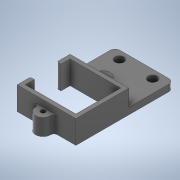
# Autodesk Inventor part: SocketMount
Saved by Autodesk Inventor 2020.2 (Build 242310000, 310)
## iProperties
Created: 2020-08-26
Part Number: SocketMount
Material: Generic
Document SubType Name: Modeling
Designer: JK
Density: 1 g/cm^3
Appearance: Smooth - Black
Author: JK
Autodesk Inventor part; units mm, degrees
ref_plane "YZ Plane" through (0, 0, 0) normal (1, 0, 0) x (0, 1, 0)
ref_plane "XZ Plane" through (0, 0, 0) normal (0, 1, 0) x (-1, 0, 0)
ref_plane "XY Plane" through (0, 0, 0) normal (0, 0, 1) x (1, 0, 0)
sketch "Sketch1" plane through (0, 0, 0) normal (0, 1, 0) x (-1, 0, 0)
  line L0 (-26.4056, 15.9) -> (8.8944, 15.9)
  line L1 (8.8944, 15.9) -> (8.8944, -15.9)
  line L2 (8.8944, -15.9) -> (-26.4056, -15.9)
  line L3 (-26.4056, -15.9) -> (-26.4056, 15.9)
  line L4 (6.4944, 13.5) -> (-24.0056, 13.5)
  line L5 (-24.0056, 13.5) -> (-24.0056, -13.5)
  line L6 (-24.0056, -13.5) -> (6.4944, -13.5)
  line L7 (6.4944, -13.5) -> (6.4944, 13.5)
  point P0 (0, 0)
  dimension "d4" = 27
  dimension "d5" = 30.5
  dimension "d7" = 2.4
  dimension "d8" = 2.4
  dimension "d9" = 2.4
  dimension "d10" = 2.4
  constraints: 16 end point, 4 parallel, 2 horizontal, 2 perpendicular
  measures "d4" distance of L6.end L4.start
  measures "d5" distance of L5.end L6.end
  measures "d7" distance between parallel lines of L1 L7
  measures "d8" distance between parallel lines of L2 L6
  measures "d9" distance between parallel lines of L3 L5
  measures "d10" distance between parallel lines of L0 L4
extrude "Extrusion1" add sketch "Sketch1" along normal blind 14
sketch "Sketch2" plane through (0, 0, 0) normal (0, -1, 0) x (1, 0, 0)
  circle A0 centre (8.7556, 18) radius 1.4
  circle A1 centre (8.7556, -18) radius 1.4
  line L0 (24.0056, -13.5) -> (24.0056, 13.5) projected
  circle A2 centre (8.7556, 18) radius 4.5
  circle A3 centre (8.7556, -18) radius 4.5
  line L1 (-6.4944, -13.5) -> (24.0056, -13.5) projected
  point P0 (0, 0)
  dimension "d13" = 36
  dimension "d14" = 15.25
  dimension "d15" = 2.8
  dimension "d16" = 18
  constraints: 4 centre point, 2 coincident, 2 equal radius, 1 tangent, 1 vertical alignment
  measures "d13" distance of A1.centre A0.centre
  measures "d14" distance from line of A0.centre L0
  measures "d15" diameter of A0
  measures "d16" vertical distance of A0.centre point (0, 0)
extrude "Extrusion2" add sketch "Sketch2" against normal blind 10
fillet "Fillet1" radius 2 4 edges at (12.7355, 5, -15.9) (4.7756, 5, -15.9) (4.7756, 5, 15.9) (12.7355, 5, 15.9)
sketch "Sketch3" plane through (0, 0, 0) normal (0, -1, 0) x (1, 0, 0)
  circle A0 centre (8.7556, -18) radius 1.4 projected
  circle A1 centre (8.7556, 18) radius 1.4 projected
  line L0 (26.4056, -15.9) -> (15.2548, -15.9) projected
  line L1 (26.4056, 15.9) -> (26.4056, -15.9) projected
  line L2 (15.2548, 15.9) -> (26.4056, 15.9) projected
  arc A2 (13.255, 17.9308) -> (15.2548, 15.9) centre (15.2548, 17.9) ccw projected
  arc A3 (13.255, 17.9308) -> (4.2561, 17.9308) centre (8.7556, 18) ccw projected
  arc A4 (2.2563, 15.9) -> (4.2561, 17.9308) centre (2.2563, 17.9) ccw projected
  line L3 (-8.8944, 15.9) -> (2.2563, 15.9) projected
  line L4 (-8.8944, -15.9) -> (-8.8944, 15.9) projected
  line L5 (2.2563, -15.9) -> (-8.8944, -15.9) projected
  arc A5 (4.2561, -17.9308) -> (2.2563, -15.9) centre (2.2563, -17.9) ccw projected
  arc A6 (4.2561, -17.9308) -> (13.255, -17.9308) centre (8.7556, -18) ccw projected
  arc A7 (15.2548, -15.9) -> (13.255, -17.9308) centre (15.2548, -17.9) ccw projected
  line L6 (-6.4944, -13.5) -> (24.0056, -13.5) projected
  line L7 (-6.4944, 13.5) -> (-6.4944, -13.5) projected
  line L8 (24.0056, 13.5) -> (-6.4944, 13.5) projected
  line L9 (24.0056, -13.5) -> (24.0056, 13.5) projected
  line L10 (26.4056, 15.9) -> (26.4056, -15.9) projected
  line L11 (26.4056, -15.9) -> (-8.8944, -15.9)
  line L12 (-8.8944, -15.9) -> (-8.8944, -43)
  line L13 (-8.8944, -43) -> (26.4056, -43)
  line L14 (26.4056, -43) -> (26.4056, -15.9)
  circle A8 centre (18.7556, -38) radius 2.75
  circle A9 centre (-1.2444, -38) radius 2.75
  line L15 (-8.8944, -15.9) -> (-8.8944, 15.9) projected
  point P0 (0, 0)
  dimension "d20" = 5.5
  dimension "d21" = 20
  dimension "d22" = 20
  dimension "d23" = 5
  dimension "d25" = 10
  constraints: 8 end point, 2 centre point, 2 parallel, 1 collinear, 1 equal radius, 1 horizontal, 1 horizontal alignment, 1 perpendicular
  measures "d20" diameter of A8
  measures "d21" vertical distance of A0.centre A9.centre
  measures "d22" distance of A8.centre A9.centre
  measures "d23" distance from line of L13 A8.centre
  measures "d25" horizontal distance of A0.centre A8.centre
extrude "Extrusion3" add sketch "Sketch3" against normal blind 4 contours L14 L13 L12 L5 A5 A6 A7 L0
fillet "Fillet2" radius 3 2 edges at (26.4056, 2, -43) (-8.8944, 2, -43)
sketch "Sketch4" plane through (0, 14, 0) normal (0, 1, 0) x (1, 0, 0)
  line L0 (-1.1926, 8) -> (-11.7963, 8)
  line L1 (-11.7963, 8) -> (-11.7963, -8)
  line L2 (-11.7963, -8) -> (-1.1926, -8)
  line L3 (-1.1926, -8) -> (-1.1926, 8)
  line L4 (-6.4944, -13.5) -> (-6.4944, 13.5) projected
  line L5 (-1.1926, 8) -> (-11.7963, -8) construction
  line L6 (-11.7963, 8) -> (-1.1926, -8) construction
  point P0 (0, 0)
  point P1 (-6.4944, 0)
  dimension "d29" = 8
  constraints: 12 end point, 3 midpoint, 2 parallel, 1 horizontal, 1 perpendicular
  measures "d29" distance from line of point (-6.494, 0) L0
extrude "Extrusion4" cut sketch "Sketch4" against normal through all
fillet "Fillet3" radius 1 2 edges at (-8.8944, 7, -8) (-8.8944, 7, 8)
body "Solid1"
